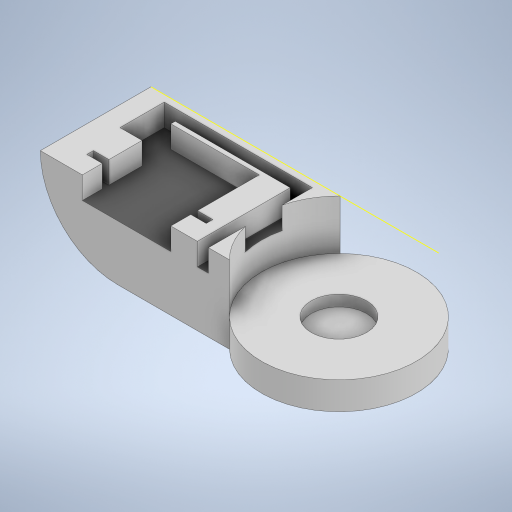
# Autodesk Inventor part: wirst 2 left
Saved by Autodesk Inventor 2023 (Build 270158000, 158)
## iProperties
Created: 2024-06-28
Part Number: wirst 2 left
Material: Generic
Document SubType Name: Modeling
Designer: Swoby
Density: 1 g/cm^3
Appearance: Default
Author: Swoby
Autodesk Inventor part; units mm, degrees
ref_plane "YZ Plane" through (0, 0, 0) normal (1, 0, 0) x (0, 1, 0)
ref_plane "XZ Plane" through (0, 0, 0) normal (0, 1, 0) x (-1, 0, 0)
ref_plane "XY Plane" through (0, 0, 0) normal (0, 0, 1) x (1, 0, 0)
sketch "Sketch1" plane through (0, 0, 0) normal (0, 0, 1) x (1, 0, 0)
  line L0 (-30, 0) -> (0, 0)
  line L1 (100, 0) -> (0, 0)
  line L2 (100, 0) -> (100, -35)
  line L3 (100, -35) -> (5, -35)
  arc A0 (-30, 0) -> (5, -35) centre (5, 0) ccw
  dimension "d0" = 30
  dimension "d26" = 130
  dimension "d27" = 35
  dimension "d28" = 35
  constraints: 8 end point, 2 point on circle, 1 centre point, 1 collinear, 1 horizontal, 1 perpendicular, 1 tangent, 1 vertical
  measures "d0" distance of L0.start L0.end
  measures "d26" distance from line of L2 L0.start
  measures "d27" distance of L1.start L2.end
  measures "d28" horizontal distance of L0.start L3.end
extrude "Extrusion1" add sketch "Sketch1" against normal blind 50
sketch "Sketch2" plane through (-30, 0, 0) normal (0, 1, 0) x (1, 0, 0)
  circle A0 centre (110, 25) radius 12.5
  circle A1 centre (110, 25) radius 35
  line L0 (0, 0) -> (0, 50) projected
  line L1 (0, 25) -> (130, 25)
  line L2 (130, 0) -> (130, 50) projected
  point P0 (30, 0)
  dimension "d6" = 25
  dimension "d7" = 70
  dimension "d8" = 110
  constraints: 2 centre point, 2 end point, 2 midpoint, 1 coincident, 1 point on line
  measures "d6" diameter of A0
  measures "d7" diameter of A1
  measures "d8" distance from line of L0 A0.centre
sketch "Sketch3" plane through (-30, 0, 0) normal (0, 1, 0) x (1, 0, 0)
  line L0 (0, 50) -> (130, 50) projected
extrude "Extrusion4" add sketch "Sketch2" against normal up to surface (35 mm away) contours L1 A0 | A0 L1 | A1
sketch "Sketch4" plane through (-30, 0, 0) normal (0, 1, 0) x (1, 0, 0)
  line L0 (85.5051, 0) -> (0, 0) projected
  line L1 (19, 0) -> (19, 9)
  line L2 (19, 9) -> (12, 9)
  line L3 (12, 9) -> (12, 12)
  line L4 (12, 12) -> (19, 12)
  line L5 (19, 12) -> (19, 27)
  line L6 (19, 27) -> (9, 27)
  line L7 (9, 27) -> (9, 47)
  line L8 (9, 47) -> (76, 47)
  line L9 (76, 47) -> (76, 0)
  line L10 (71, 0) -> (71, 42)
  line L11 (71, 42) -> (19, 42)
  line L12 (19, 42) -> (19, 40)
  line L13 (19, 40) -> (59, 40)
  line L14 (59, 40) -> (59, 12)
  line L15 (59, 12) -> (66, 12)
  line L16 (66, 12) -> (66, 9)
  line L17 (66, 9) -> (59, 9)
  line L18 (59, 9) -> (59, 0)
  point P0 (30, 0)
  point P1 (12, 10.5)
  point P2 (66, 10.5)
  dimension "d31" = 54
  dimension "d32" = 36
  dimension "d33" = 7
  dimension "d34" = 7
  dimension "d35" = 40
  dimension "d36" = 2
  dimension "d37" = 3
  dimension "d38" = 9
  dimension "d39" = 15
  dimension "d40" = 10
  dimension "d41" = 20
  dimension "d42" = 5
  dimension "d43" = 67
  constraints: 36 end point, 11 perpendicular, 8 point on line, 3 collinear, 2 midpoint, 2 vertical, 1 horizontal, 1 parallel
  measures "d31" distance from line of point (12, 10.5) L16
  measures "d32" horizontal distance of point (66, 10.5) point (30, 0)
  measures "d33" distance of L1.end L2.end
  measures "d34" distance of L16.end L17.end
  measures "d35" distance between parallel lines of L13 L0
  measures "d36" distance of L11.end L12.end
  measures "d37" distance of L2.end L3.end
  measures "d38" distance of L1.start L1.end
  measures "d39" distance of L4.end L5.end
  measures "d40" distance between parallel lines of L5 L7
  measures "d41" distance of L6.end L7.end
  measures "d42" distance between parallel lines of L10 L9
  measures "d43" distance of L7.end L8.end
extrude "Extrusion5" cut sketch "Sketch4" against normal blind 10 contours L0 L10 L11 L12 L13 L14 L15 L16 L17 L18 L1 L2 L3 L4 L5 L6 L7 L8 L9
sketch "Sketch5" plane through (-30, 0, 0) normal (0, 1, 0) x (1, 0, 0)
  arc A0 (85.5051, 0) -> (85.5051, 50) centre (110, 25) ccw projected
  circle A1 centre (110, 25) radius 35
  circle A2 centre (110, 25) radius 12.5
  point P0 (30, 0)
  point P1 (85.5051, 50)
  point P2 (85.5051, 0)
  dimension "d46" = 25
  constraints: 2 centre point, 2 coincident, 1 concentric
  measures "d46" diameter of A2
extrude "Extrusion6" cut sketch "Sketch5" against normal blind 22.5 contours A1 A0 | A2
sketch "Sketch6" plane through (-30, -22.5, 0) normal (0, 1, 0) x (1, 0, 0)
  arc A0 (85.5051, 0) -> (85.5051, 50) centre (110, 25) ccw projected
  arc A1 (85.5051, 50) -> (85.5051, 0) centre (110, 25) ccw projected
  circle A2 centre (110, 25) radius 12.5
  point P0 (30, 0)
  dimension "d49" = 25
  constraints: 1 centre point, 1 coincident
  measures "d49" diameter of A2
extrude "Extrusion7" cut sketch "Sketch6" against normal blind 5 contours A2
body "Solid1"
